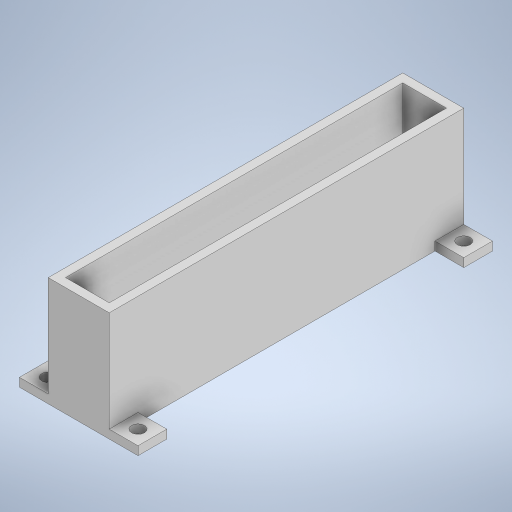
# Autodesk Inventor part: HDD_fastening
Saved by Autodesk Inventor 2024 (Build 280153000, 153)
## iProperties
Created: 2024-05-18
Part Number: HDD_fastening
Material: Generic
Document SubType Name: Modeling
Designer: inigo
Density: 1 g/cm^3
Appearance: Default
Author: inigo
Autodesk Inventor part; units mm, degrees
ref_plane "YZ Plane" through (0, 0, 0) normal (1, 0, 0) x (0, 1, 0)
ref_plane "XZ Plane" through (0, 0, 0) normal (0, 1, 0) x (-1, 0, 0)
ref_plane "XY Plane" through (0, 0, 0) normal (0, 0, 1) x (1, 0, 0)
sketch "Sketch1" plane through (0, 0, 0) normal (0, 1, 0) x (-1, 0, 0)
  line L0 (7.6, 58.6) -> (-7.6, 58.6)
  line L1 (-7.6, 58.6) -> (-7.6, -58.6)
  line L2 (-7.6, -58.6) -> (7.6, -58.6)
  line L3 (7.6, -58.6) -> (7.6, 58.6)
  line L4 (7.6, 58.6) -> (-7.6, -58.6) construction
  line L5 (-7.6, 58.6) -> (7.6, -58.6) construction
  line L6 (10.6, 61.6) -> (-10.6, 61.6)
  line L7 (-10.6, 61.6) -> (-10.6, -61.6)
  line L8 (-10.6, -61.6) -> (10.6, -61.6)
  line L9 (10.6, -61.6) -> (10.6, 61.6)
  point P0 (0, 0)
  dimension "d0" = 15.2
  dimension "d1" = 117.2
  dimension "d2" = 3
  constraints: 20 end point, 4 parallel, 2 midpoint, 2 perpendicular, 1 horizontal, 3 other
  measures "d0" distance of L2.end L1.end
  measures "d1" distance of L1.end L0.end
  measures "d2" distance between parallel lines of L3 L9
extrude "Extrusion1" add sketch "Sketch1" along normal blind 35
sketch "Sketch2" plane through (0, 0, 0) normal (0, -1, 0) x (1, 0, 0)
  circle A0 centre (15.6, 56.6) radius 2.25
  line L0 (10.6, 61.6) -> (10.6, -61.6) projected
  line L1 (-10.6, 61.6) -> (10.6, 61.6) projected
  line L2 (10.6, 0) -> (40.0952, 0)
  line L3 (10.6, -61.6) -> (-10.6, -61.6) projected
  line L4 (0, -61.6) -> (0, -71.4925)
  line L5 (10.6, 61.6) -> (20.6, 61.6)
  line L6 (20.6, 61.6) -> (20.6, 51.6)
  line L7 (20.6, 51.6) -> (10.6, 51.6)
  line L8 (10.6, 51.6) -> (10.6, 61.6)
  line L9 (-10.6, 61.6) -> (10.6, 61.6)
  line L10 (10.6, 61.6) -> (10.6, -61.6)
  line L11 (10.6, -61.6) -> (-10.6, -61.6)
  line L12 (-10.6, -61.6) -> (-10.6, 61.6)
  circle A1 centre (15.6, -56.6) radius 2.25
  line L13 (10.6, -61.6) -> (20.6, -61.6)
  line L14 (20.6, -61.6) -> (20.6, -51.6)
  line L15 (20.6, -51.6) -> (10.6, -51.6)
  line L16 (10.6, -51.6) -> (10.6, -61.6)
  circle A2 centre (-15.6, 56.6) radius 2.25
  line L17 (-10.6, 61.6) -> (-20.6, 61.6)
  line L18 (-20.6, 61.6) -> (-20.6, 51.6)
  line L19 (-20.6, 51.6) -> (-10.6, 51.6)
  line L20 (-10.6, 51.6) -> (-10.6, 61.6)
  line L21 (-20.6, -51.6) -> (-10.6, -51.6)
  circle A3 centre (-15.6, -56.6) radius 2.25
  line L22 (-10.6, -61.6) -> (-20.6, -61.6)
  line L23 (-20.6, -61.6) -> (-20.6, -51.6)
  line L24 (-10.6, -51.6) -> (-10.6, -61.6)
  point P0 (0, 0)
  dimension "d5" = 4.5
  dimension "d6" = 5
  dimension "d7" = 5
  dimension "d8" = 5
  dimension "d9" = 5
  constraints: 44 end point, 19 symmetric about line, 4 centre point, 4 parallel, 3 horizontal, 2 midpoint, 2 perpendicular, 1 vertical, 3 other
  measures "d5" diameter of A0
  measures "d6" distance from line of L0 A0.centre
  measures "d7" distance from line of A0.centre L1
  measures "d8" distance from line of L7 A0.centre
  measures "d9" distance from line of A0.centre L6
extrude "Extrusion2" add sketch "Sketch2" along normal blind 3
body "Solid1"
